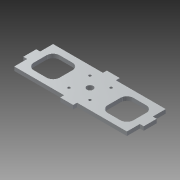
# Autodesk Inventor part: OpenROV 2_3 Dev Vertical Motor Mount
Saved by Autodesk Inventor 2015 (Build 190159000, 159)
## iProperties
Created: 2012-05-11
Part Number: OpenROV 2_3 Dev Vertical Motor Mount
Material: Generic
Document SubType Name: Modeling
Designer: user
Density: 1 g/cm^3
Appearance: Default
Author: user
Autodesk Inventor part; units mm, degrees
ref_plane "YZ Plane" through (0, 0, 0) normal (1, 0, 0) x (0, 1, 0)
ref_plane "XZ Plane" through (0, 0, 0) normal (0, 1, 0) x (-1, 0, 0)
ref_plane "XY Plane" through (0, 0, 0) normal (0, 0, 1) x (1, 0, 0)
sketch "Sketch1" plane through (0, 0, 0) normal (0, 0, 1) x (1, 0, 0)
  line L0 (0, 0) -> (0, 10)
  line L1 (0, 10) -> (-3, 10)
  line L2 (-3, 10) -> (-3, 20)
  line L3 (-3, 20) -> (0, 20)
  line L4 (0, 20) -> (0, 30)
  line L5 (0, 30) -> (38.5, 30)
  line L6 (38.5, 30) -> (38.5, 33)
  line L7 (38.5, 33) -> (48.5, 33)
  line L8 (48.5, 33) -> (48.5, 30)
  line L9 (48.5, 30) -> (87, 30)
  line L10 (87, 30) -> (87, 20)
  line L11 (87, 20) -> (90, 20)
  line L12 (90, 20) -> (90, 10)
  line L13 (90, 10) -> (87, 10)
  line L14 (87, 10) -> (87, 0)
  line L15 (87, 0) -> (48.5, 0)
  line L16 (48.5, 0) -> (48.5, -3)
  line L17 (48.5, -3) -> (38.5, -3)
  line L18 (38.5, -3) -> (38.5, 0)
  line L19 (38.5, 0) -> (0, 0)
  line L20 (10, 25) -> (20, 25)
  line L21 (25, 20) -> (25, 10)
  line L22 (20, 5) -> (10, 5)
  line L23 (5, 10) -> (5, 20)
  line L24 (67, 25) -> (77, 25)
  line L25 (82, 20) -> (82, 10)
  line L26 (77, 5) -> (67, 5)
  line L27 (62, 10) -> (62, 20)
  arc A0 (10, 25) -> (5, 20) centre (10, 20) ccw
  arc A1 (25, 20) -> (20, 25) centre (20, 20) ccw
  arc A2 (20, 5) -> (25, 10) centre (20, 10) ccw
  arc A3 (5, 10) -> (10, 5) centre (10, 10) ccw
  arc A4 (67, 25) -> (62, 20) centre (67, 20) ccw
  arc A5 (82, 20) -> (77, 25) centre (77, 20) ccw
  arc A6 (77, 5) -> (82, 10) centre (77, 10) ccw
  arc A7 (62, 10) -> (67, 5) centre (67, 10) ccw
  circle A8 centre (43.5, 15) radius 2.5
  circle A9 centre (35.3683, 23.1317) radius 1
  circle A10 centre (35.3683, 6.8683) radius 1
  circle A11 centre (51.6317, 6.8683) radius 1
  circle A12 centre (51.6317, 23.1317) radius 1
  dimension "d0" = 10
  dimension "d1" = 10
  dimension "d2" = 10
  dimension "d3" = 10
  dimension "d4" = 10
  dimension "d5" = 10
  dimension "d6" = 38.5
  dimension "d7" = 38.5
  dimension "d8" = 10
  dimension "d9" = 38.5
  dimension "d11" = 38.5
  dimension "d12" = 5
  dimension "d13" = 5
  dimension "d15" = 5
  dimension "d16" = 20
  dimension "d17" = 5
  dimension "d18" = 5
  dimension "d19" = 5
  dimension "d20" = 20
  dimension "d21" = 3
  dimension "d23" = 3
  dimension "d24" = 3
  dimension "d25" = 5
  dimension "d26" = 5
  dimension "d27" = 5
  dimension "d28" = 15
  dimension "d30" = 2
  dimension "d34" = 360
  dimension "d38" = 3
  dimension "d39" = 10
  constraints: 56 end point, 20 parallel, 16 point on circle, 16 tangent, 13 centre point, 7 equal radius, 3 perpendicular, 2 collinear, 2 horizontal, 1 horizontal alignment, 1 vertical, 1 vertical alignment, 9 other
  measures "d0" distance between parallel lines of L19 L1
  measures "d1" distance of L1.end L2.end
  measures "d2" distance of L3.end L4.end
  measures "d3" distance of L9.end L10.end
  measures "d4" distance of L11.end L12.end
  measures "d5" distance of L13.end L14.end
  measures "d6" distance of L4.end L5.end
  measures "d7" distance of L8.end L9.end
  measures "d8" distance of L6.end L7.end
  measures "d9" distance of L14.end L15.end
  measures "d11" distance of L18.end L0.start
  measures "d12" distance between parallel lines of L23 L4
  measures "d13" distance between parallel lines of L5 L20
  measures "d15" distance between parallel lines of L19 L22
  measures "d16" distance between parallel lines of L23 L21
  measures "d17" distance between parallel lines of L9 L24
  measures "d18" distance between parallel lines of L10 L25
  measures "d19" distance between parallel lines of L15 L26
  measures "d20" distance between parallel lines of L27 L25
  measures "d21" distance between parallel lines of L5 L7
  measures "d23" distance between parallel lines of L0 L2
  measures "d24" distance between parallel lines of L14 L12
  measures "d25" radius of A0
  measures "d26" diameter of A8
  measures "d27" distance from line of A8.centre L8
  measures "d28" distance from line of L15 A8.centre
  measures "d30" diameter of A9
  measures "d38" distance between parallel lines of L19 L17
  measures "d39" distance of L16.end L17.end
extrude "Extrusion1" add sketch "Sketch1" along normal blind 3
body "Solid1"
